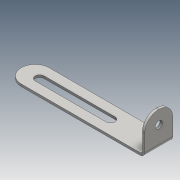
# Autodesk Inventor part: apoio de escudo
Saved by Autodesk Inventor 2016 (Build 200138000, 138)
## iProperties
Created: 2018-10-22
Part Number: apoio de escudo
Material: Genérico
Document SubType Name: Sheet Metal
Designer: thiag
Density: 1 g/cm^3
Appearance: Padrão
Sheet Metal Rule: Default
Author: thiag
Autodesk Inventor part; units mm, degrees
ref_plane "YZ Plane" through (0, 0, 0) normal (1, 0, 0) x (0, 1, 0)
ref_plane "XZ Plane" through (0, 0, 0) normal (0, 1, 0) x (-1, 0, 0)
ref_plane "XY Plane" through (0, 0, 0) normal (0, 0, 1) x (1, 0, 0)
sketch "Esboço1" plane through (0, 0, 0) normal (0, 0, 1) x (1, 0, 0)
  line L0 (-18.5827, 6.5782) -> (32.5173, 6.5782)
  line L1 (-18.5827, -4.9718) -> (32.5173, -4.9718)
  line L2 (32.5173, -4.9718) -> (32.5173, 6.5782)
  arc A0 (-18.5827, 6.5782) -> (-18.5827, -4.9718) centre (-18.5827, 0.8032) ccw
  line L3 (-16.7327, 2.6532) -> (12.5673, 2.6532)
  line L4 (12.5673, -1.0468) -> (-16.7327, -1.0468)
  arc A1 (-16.7327, 2.6532) -> (-16.7327, -1.0468) centre (-16.7327, 0.8032) ccw
  arc A2 (12.5673, -1.0468) -> (12.5673, 2.6532) centre (12.5673, 0.8032) ccw
  point P0 (0, 0)
  point P1 (-2.0827, 0.8032)
  point P2 (-2.0827, 0.8032)
  constraints: 10 end point, 6 point on circle, 4 tangent, 3 centre point, 2 horizontal, 1 parallel, 1 perpendicular
extrude "Extrusão1" add sketch "Esboço1" along normal blind 1
sketch "Esboço2" plane through (0, 0, 1) normal (0, 0, 1) x (1, 0, 0)
  line L0 (32.5173, 6.5782) -> (31.5173, 6.5782)
  line L1 (31.5173, 6.5782) -> (31.5173, -4.9718)
  line L2 (31.5173, -4.9718) -> (32.5173, -4.9718)
  line L3 (32.5173, -4.9718) -> (32.5173, 6.5782)
  point P0 (0, 0)
  dimension "d8" = 1
  constraints: 8 end point, 2 parallel, 1 horizontal, 1 perpendicular
  measures "d8" distance of L2.end L1.end
extrude "Extrusão2" add sketch "Esboço2" along normal blind 13.5
fillet "Arredondamento1" radius 5.5 1 edges at (32.0173, 6.5782, 14.5)
fillet "Arredondamento2" radius 5.5 1 edges at (32.0173, -4.9718, 14.5)
sketch "Esboço3" plane through (32.5173, -4.9718, 0) normal (1, 0, 0) x (0, 0, -1)
  circle A0 centre (-9, 5.775) radius 1.5
  point P0 (0, 4.9718)
  constraints: 1 centre point
hole "Furo1" at (32.5173, 0.8032, 9) direction (-1, 0, 0) diameter 3 end through all
fillet "Fillet3" radius 0.7 1 edges at (31.5173, 0.8032, 1)
fillet "Fillet4" radius 2 1 edges at (32.5173, 0.8032, 0)
equation "\"BendRadius\" = Thickness"
equation "\"BendReliefWidth\" = Thickness"
equation "\"BendReliefDepth\" = 0.5 * Thickness"
equation "\"CornerReliefSize\" = 4 * Thickness"
equation "\"MinimumRemnant\" = 2 * Thickness"
equation "\"TransitionRadius\" = BendRadius"
equation "\"JacobiRadiusSize\" = Thickness"
equation "\"GapSize\" = Thickness"
equation "\"Thickness\" = 0.5"
